e6e0dd21-42b0-41c0-abb6-053d1b85874a (Autodesk Fusion 360 design; units mm, degrees)
Autodesk Fusion 360 part; units mm, degrees
sketch "Sketch1" plane through (0, 0, 0) normal (0, 1, 0) x (1, 0, 0)
  circle A0 centre (0, 0) radius 12.7
  circle A1 centre (0, 0) radius 13.716
  circle A2 centre (0, 0) radius 11.6417
  circle A3 centre (0, 0) radius 11.9341
  arc A4 (13.6809, -0.9813) -> (-12.5718, -5.4845) centre (0, 0) ccw
  circle A5 centre (0, 0) radius 4.7625
  line L0 (0, 0) -> (13.716, 0) construction
  line L1 (0, 0) -> (-1.0401, -11.8887)
  line L2 (0, 0) -> (-2.0723, -11.7528)
  line L3 (0, 0) -> (-3.0888, -11.5275)
  line L4 (0, 0) -> (-4.0817, -11.2144)
  line L5 (0, 0) -> (-5.0436, -10.816)
  line L6 (0, 0) -> (-5.967, -10.3352)
  line L7 (0, 0) -> (-6.8451, -9.7758)
  line L8 (-1.0401, -11.8887) -> (-0.0026, -11.9795) construction
  line L9 (-2.0723, -11.7528) -> (-0.0211, -12.1145) construction
  line L10 (-3.0888, -11.5275) -> (-0.0709, -12.3361) construction
  line L11 (-4.0817, -11.2144) -> (-0.1671, -12.6392) construction
  line L12 (-5.0436, -10.816) -> (-0.3242, -13.0166) construction
  line L13 (-5.967, -10.3352) -> (-0.5555, -13.4596) construction
  line L14 (-6.8451, -9.7758) -> (-0.8734, -13.9573) construction
  line L15 (0, 0) -> (-7.6711, -9.142)
  line L16 (-7.6711, -9.142) -> (-1.2887, -14.4975) construction
  line L17 (0, 0) -> (-8.4387, -8.4387)
  line L18 (-8.4387, -8.4387) -> (-1.811, -15.0664) construction
  spline S0 degree 5 poles (-1.811, -15.0664) (-1.7953, -15.0464) (-1.7637, -15.0068) (-1.7154, -14.949) (-1.6495, -14.8746) (-1.5653, -14.7853) (-1.4808, -14.6986) (-1.3971, -14.6132) (-1.3156, -14.5277) (-1.2373, -14.4413) (-1.1627, -14.3535) (-1.0918, -14.2644) (-1.0243, -14.1743) (-0.9598, -14.0838) (-0.8977, -13.9936) (-0.8374, -13.9041) (-0.7788, -13.8157) (-0.7219, -13.7284) (-0.6668, -13.6423) (-0.6137, -13.5572) (-0.5628, -13.4728) (-0.5144, -13.3891) (-0.4686, -13.3061) (-0.4252, -13.224) (-0.3842, -13.1428) (-0.3455, -13.0628) (-0.309, -12.9843) (-0.2746, -12.9074) (-0.2422, -12.8321) (-0.2121, -12.7584) (-0.1842, -12.6865) (-0.1586, -12.6165) (-0.1352, -12.5484) (-0.1139, -12.4825) (-0.0945, -12.4193) (-0.077, -12.3588) (-0.0612, -12.3013) (-0.0474, -12.2469) (-0.0356, -12.1953) (-0.0261, -12.1468) (-0.0188, -12.1015) (-0.0133, -12.06) (-0.0089, -12.0235) (-0.0049, -11.993) (-0.0011, -11.9693) (0.0021, -11.9522) (0.003, -11.9429) (0.0022, -11.9378) (0.0009, -11.9352) (0, -11.9341) knots 0 0 0 0 0 0 0.022222 0.044444 0.066667 0.088889 0.111111 0.133333 0.155556 0.177778 0.2 0.222222 0.244444 0.266667 0.288889 0.311111 0.333333 0.355556 0.377778 0.4 0.422222 0.444444 0.466667 0.488889 0.511111 0.533333 0.555556 0.577778 0.6 0.622222 0.644444 0.666667 0.688889 0.711111 0.733333 0.755556 0.777778 0.8 0.822222 0.844444 0.866667 0.888889 0.911111 0.933333 0.955556 0.977778 1 1 1 1 1 1
  line L19 (-1.9066, -15.1886) -> (-1.7153, -14.9442)
  line L20 (0.0421, -11.9886) -> (-0.0421, -11.8796)
  line L21 (-0.1892, -12.6986) -> (0, 0)
  line L22 (0, 0) -> (-0.4932, -6.1248) construction
  line L23 (0, -11.9341) -> (0, 0) construction
  spline S1 degree 5 poles (0, -11.9341) (0, -11.9142) (0, -11.8779) (0, -11.8346) (0, -11.7947) (0, -11.7574) (0, -11.7229) (0, -11.6871) (0, -11.6577) (0, -11.6417) knots 0 0 0 0 0 0 0.2 0.4 0.6 0.8 1 1 1 1 1 1
  spline S2 degree 5 poles (-1.9095, -11.7803) (-1.9063, -11.7606) (-1.9005, -11.7249) (-1.8936, -11.6821) (-1.8872, -11.6427) (-1.8812, -11.6059) (-1.8757, -11.5718) (-1.87, -11.5365) (-1.8653, -11.5075) (-1.8627, -11.4917) knots 0 0 0 0 0 0 0.2 0.4 0.6 0.8 1 1 1 1 1 1
  line L24 (0, -12.0222) -> (0, -11.846)
  line L25 (0, -11.7127) -> (0, -11.5706)
  line L26 (-1.9236, -11.8673) -> (-1.8954, -11.6934)
  line L27 (-1.8741, -11.5618) -> (-1.8514, -11.4216)
  spline S3 degree 5 poles (-0.6231, -15.1621) (-0.6353, -15.1398) (-0.6602, -15.0957) (-0.6986, -15.0308) (-0.7518, -14.9468) (-0.8206, -14.8453) (-0.8902, -14.7462) (-0.9591, -14.6484) (-1.0259, -14.5511) (-1.0894, -14.4532) (-1.149, -14.3546) (-1.2047, -14.2553) (-1.2568, -14.1556) (-1.3061, -14.0559) (-1.353, -13.9569) (-1.3981, -13.8589) (-1.4418, -13.7623) (-1.484, -13.6671) (-1.5247, -13.5733) (-1.5635, -13.4807) (-1.6002, -13.3893) (-1.6345, -13.2989) (-1.6665, -13.2097) (-1.6962, -13.1216) (-1.7236, -13.0349) (-1.749, -12.9498) (-1.7726, -12.8665) (-1.7942, -12.785) (-1.8141, -12.7055) (-1.832, -12.628) (-1.848, -12.5526) (-1.8621, -12.4793) (-1.8743, -12.4083) (-1.8848, -12.3399) (-1.8938, -12.2744) (-1.9015, -12.2119) (-1.9078, -12.1526) (-1.9128, -12.0967) (-1.9162, -12.0439) (-1.9178, -11.9945) (-1.9178, -11.9486) (-1.9165, -11.9067) (-1.915, -11.87) (-1.9141, -11.8393) (-1.9141, -11.8153) (-1.9145, -11.7979) (-1.9139, -11.7885) (-1.9123, -11.7836) (-1.9105, -11.7813) (-1.9095, -11.7803) knots 0 0 0 0 0 0 0.022222 0.044444 0.066667 0.088889 0.111111 0.133333 0.155556 0.177778 0.2 0.222222 0.244444 0.266667 0.288889 0.311111 0.333333 0.355556 0.377778 0.4 0.422222 0.444444 0.466667 0.488889 0.511111 0.533333 0.555556 0.577778 0.6 0.622222 0.644444 0.666667 0.688889 0.711111 0.733333 0.755556 0.777778 0.8 0.822222 0.844444 0.866667 0.888889 0.911111 0.933333 0.955556 0.977778 1 1 1 1 1 1
  line L28 (-0.5482, -15.298) -> (-0.6979, -15.0261)
  line L29 (-1.9598, -11.8274) -> (-1.8593, -11.7333)
  point P0 (-0.1892, -12.6986)
  point P1 (0, -11.6417)
  point P2 (-1.0475, -14.5169)
  point P3 (-1.3711, -13.9172)
  point P4 (-1.6052, -13.375)
  point P5 (-1.7627, -12.9008)
  point P6 (-1.8574, -12.5031)
  point P7 (-1.9039, -12.1885)
  point P8 (-1.9176, -11.9618)
  point P9 (-1.9142, -11.8255)
  point P10 (-1.8627, -11.4917)
  dimension "d2" = 27.432
  dimension "id" = 23.2833
  dimension "BaseDiameter" = 23.8682
  dimension "d1" = 9.525
  dimension "d34" = 5
  dimension "d35" = 5
  dimension "d36" = 5
  dimension "d37" = 5
  dimension "d38" = 5
  dimension "d39" = 5
  dimension "d41" = 1.0414
  dimension "d42" = 2.0829
  dimension "d43" = 3.1243
  dimension "d44" = 4.1658
  dimension "d45" = 5.2072
  dimension "d46" = 6.2487
  dimension "d47" = 7.2901
  dimension "d48" = 5
  dimension "d49" = 8.3316
  dimension "d50" = 5
  dimension "d51" = 9.373
  dimension "d55" = 3.75
  dimension "d60" = 5
  constraint coincident A0.centre A1.centre
  constraint concentric A0 A2
  constraint coincident A1 A4.end
  constraint horizontal L0
  constraint coincident A4 L0.end
  constraint coincident A3 S0.end
  constraint coincident A3 L1.end
  constraint coincident A3 L2.end
  constraint coincident A3 L3.end
  constraint coincident A3 L4.end
  constraint coincident A3 L5.end
  constraint coincident A3 L6.end
  constraint coincident A3 L7.end
  constraint vertical A0.centre S0.end
  constraint tangent A3 L8
  constraint tangent A3 L9
  constraint tangent A3 L10
  constraint tangent A3 L11
  constraint tangent A3 L12
  constraint tangent A3 L13
  constraint tangent A3 L14
  constraint coincident A3 L15.end
  constraint tangent A3 L16
  constraint coincident A3 L17.end
  constraint tangent A3 L18
  constraint midpoint L18.end L19
  constraint midpoint S0.end L20
  constraint coincident A0 P0
  constraint coincident S0 P0
  constraint coincident P0 L21.start
  constraint coincident L23 P1
  constraint coincident A2 P1
  constraint coincident P1 S1.end
  constraint midpoint S0.end L24
  constraint midpoint P1 L25
  constraint symmetric S0.end L22 S2.start
  constraint symmetric L8.end L22 P9
  constraint symmetric L9.end L22 P8
  constraint symmetric L10.end L22 P7
  constraint symmetric L11.end L22 P6
  constraint symmetric L12.end L22 P5
  constraint symmetric L13.end L22 P4
  constraint symmetric L14.end L22 P3
  constraint symmetric L16.end L22 P2
  constraint symmetric L18.end L22 S3.start
  constraint symmetric L19.start L22 L28.start
  constraint symmetric L19.end L22 L28.end
  constraint symmetric L20.start L22 L29.start
  constraint symmetric L20.end L22 L29.end
  constraint symmetric L22 P1 P10
  constraint symmetric L22 L24.start L26.start
  constraint symmetric L22 L24.end L26.end
  constraint symmetric L22 L25.start L27.start
  constraint symmetric L22 L25.end L27.end
  constraint vertical L24
  constraint vertical L25
  measures "d2" diameter of A1
  measures "id" diameter of A2
  measures "BaseDiameter" diameter of A3
  measures "d1" diameter of A5
  measures "d34" angle of L1 L2
  measures "d35" angle of L2 L3
  measures "d36" angle of L3 L4
  measures "d37" angle of L4 L5
  measures "d38" angle of L5 L6
  measures "d39" angle of L6 L7
  measures "d41" distance of L1.end L8.end
  measures "d42" distance of L2.end L9.end
  measures "d43" distance of L3.end L10.end
  measures "d44" distance of L4.end L11.end
  measures "d45" distance of L5.end L12.end
  measures "d46" distance of L6.end L13.end
  measures "d47" distance of L7.end L14.end
  measures "d48" angle of L7 L15
  measures "d49" distance of L15.end L16.end
  measures "d50" angle of L15 L17
  measures "d51" distance of L17.end L18.end
  measures "d55" angle of L21 L22
  measures "d60" angle of L1 L23
extrude "Extrude1" add sketch "Sketch1" along normal blind 304.8 contours A0 A1 S0 S3 | A3 S0 L21 L24 | A0 A3 L21 L26 S3 | A2 A3 L21 S1 L24 L25 | A2 A3 L1 L21 | A2 A3 L1 S2 L26 L27 makes body 1
pattern_circular "C-Pattern2" count 12 over 360 about axis through (0, 1.75, 0) along (0, 1, 0) of bodies 1 makes body 2 at (5.6399, 203.2, 10.1843) makes body 3 at (9.9764, 203.2, 5.9999) makes body 4 at (11.6398, 203.2, 0.2079) makes body 5 at (10.2834, 203.2, -5.4572) makes body 6 at (5.9999, 203.2, -9.9764) makes body 7 at (0.2079, 203.2, -11.6398) makes body 8 at (-5.6399, 203.2, -10.1843) makes body 9 at (-9.9764, 203.2, -5.9999) makes body 10 at (-11.6398, 203.2, -0.2079) makes body 11 at (-10.1843, 203.2, 5.6399) makes body 12 at (-5.9999, 203.2, 9.9764)
extrude "Extrude2" add sketch "Sketch1" along normal blind 304.8 contours A2 A5 L17 L21 | A2 A5 L1 L21 | A2 A5 L1 L2 | A2 A5 L2 L3 | A2 A5 L15 L17 | A2 A5 L3 L4 | A2 A5 L4 L5 | A2 A5 L5 L6 | A2 A5 L6 L7 | A2 A5 L7 L15 bodies 1 2 3 4 5 6 7 8 9 10 11 12
ref_plane "WorkPlane1" through (6.2747, 152.4, -0.8261) normal (0.130526, 0, 0.991445) x (0.991445, 0, -0.130526)
fillet "Fillet1" [suppressed]
mirror "Mirror3" [suppressed]
pattern_circular "C-Pattern1" [suppressed]
equation "d = 1 in"
equation "OutsideDiameter = d2"
equation "PitchDiameter = d"
equation "id = PitchDiameter - 2 * ( PitchDiameter / TeethNumber )"
equation "BaseDiameter = PitchDiameter * cos(20 deg)"
equation "Length = 12 in"
equation "t = 24"
equation "ShaftDiameter = d1"
equation "TeethNumber = t"
equation "Pitch = 32"
equation "d30 = ( 1.25 * ( PitchDiameter / TeethNumber ) ) - ( PitchDiameter / TeethNumber )"
equation "Basecircum = PI * PitchDiameter * cos(20 deg)"
equation "d41 = Basecircum * 5 / 360"
equation "d42 = Basecircum * 10 / 360"
equation "d43 = Basecircum * 15 / 360"
equation "d44 = Basecircum * 20 / 360"
equation "d45 = Basecircum * 25 / 360"
equation "d46 = Basecircum * 30 / 360"
equation "d47 = Basecircum * 35 / 360"
equation "d49 = Basecircum * 40 / 360"
equation "d51 = Basecircum * 45 / 360"
equation "d55 = ( 360 / ( 4 * TeethNumber ) ) * 1 deg"
